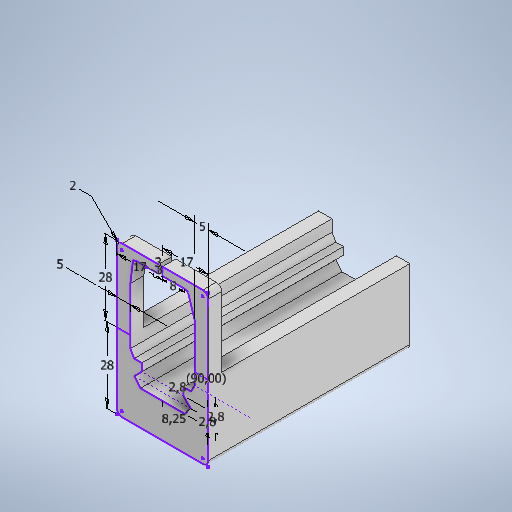
# Autodesk Inventor part: CaseV1
Saved by Autodesk Inventor 2025.2 (Build 292293000, 293)
## iProperties
Created: 2026-03-06
Part Number: CaseV1
Material: Genérico
Document SubType Name: Modeling
Designer: Periscopio
Density: 1 g/cm^3
Appearance: Valor por defecto
Author: Periscopio
Autodesk Inventor part; units mm, degrees
ref_plane "YZ Plane" through (0, 0, 0) normal (1, 0, 0) x (0, 1, 0)
ref_plane "XZ Plane" through (0, 0, 0) normal (0, 1, 0) x (-1, 0, 0)
ref_plane "XY Plane" through (0, 0, 0) normal (0, 0, 1) x (1, 0, 0)
sketch "Boceto1" plane through (0, 0, 0) normal (0, 0, 1) x (1, 0, 0)
  line L0 (0, 0) -> (8.25, 0)
  line L1 (-10.5, 2.8) -> (10.5, 2.8) construction
  line L2 (-7.75, 5.6) -> (7.75, 5.6) construction
  line L3 (10.5, 2.8) -> (8.25, 0)
  line L4 (7.75, 5.6) -> (10.5, 2.8)
  line L5 (7.75, 5.6) -> (7.75, 8.4)
  line L6 (7.75, 8.4) -> (10.55, 8.4)
  line L7 (11.95, 10.9) -> (10.55, 8.4)
  line L8 (11.95, 10.9) -> (11.95, 31.9)
  line L9 (11.95, 10.9) -> (32.95, 10.9) construction
  line L10 (9.4, 39.9) -> (11.95, 31.9)
  line L11 (9.4, 39.9) -> (9.75, 39.9) construction
  line L12 (2.95, 40.25) -> (5.95, 40.25) construction
  line L13 (0, 43.25) -> (-0.05, 43.25)
  line L14 (-3.05, 43.25) -> (-0.05, 43.25) construction
  line L15 (-0.05, 43.25) -> (-0.05, 40.25)
  line L16 (-0.05, 40.25) -> (7.95, 40.25)
  line L17 (7.95, 40.25) -> (9.4, 39.9)
  line L18 (0, 0) -> (-8.25, 0)
  line L19 (-10.5, 2.8) -> (-8.25, 0)
  line L20 (-7.75, 5.6) -> (-10.5, 2.8)
  line L21 (-7.75, 5.6) -> (-7.75, 8.4)
  line L22 (-7.75, 8.4) -> (-10.6, 8.4)
  line L23 (-12, 10.9) -> (-10.6, 8.4)
  line L24 (-12, 10.9) -> (-12, 31.9)
  line L25 (-11, 39.9) -> (-12, 31.9)
  line L26 (-11, 39.9) -> (-11.35, 39.9) construction
  line L27 (0, 43.25) -> (-1.5, 43.25)
  line L28 (-1.55, 43.25) -> (-1.55, 40.25)
  line L29 (-1.55, 40.25) -> (-9.55, 40.25)
  line L30 (-9.55, 40.25) -> (-11, 39.9)
  line L31 (-3.5, 43.25) -> (-1.5, 43.25) construction
  line L32 (0, 43.25) -> (-15, 43.25)
  line L33 (-17, 41.25) -> (-17, 15.25)
  line L34 (-17, 15.25) -> (-12, 15.25)
  line L35 (-17, 15.25) -> (-17, -10.75)
  line L36 (-15, -12.75) -> (0, -12.75)
  line L37 (16.95, 41.25) -> (16.95, 15.25)
  line L38 (16.95, 15.25) -> (11.9, 15.25)
  line L39 (16.95, 15.25) -> (16.95, -10.75)
  line L40 (14.95, -12.75) -> (0, -12.75)
  line L41 (14.95, 43.25) -> (-0.05, 43.25)
  arc A0 (-15, 43.25) -> (-17, 41.25) centre (-15, 41.25) ccw
  arc A1 (16.95, 41.25) -> (14.95, 43.25) centre (14.95, 41.25) ccw
  arc A2 (14.95, -12.75) -> (16.95, -10.75) centre (14.95, -10.75) ccw
  arc A3 (-17, -10.75) -> (-15, -12.75) centre (-15, -10.75) ccw
  point P0 (-5.95, 40.25)
  point P1 (-0.05, 43.25)
  point P2 (-17, 43.25)
  point P3 (16.95, 43.25)
  point P4 (-17, -12.75)
  point P5 (16.95, -12.75)
  point P6 (11.95, 15.25)
  point P7 (-1.55, 43.25)
  dimension "d40" = 2.8
  dimension "d45" = 90
  dimension "d52" = 8.25
  dimension "d53" = 2.8
  dimension "d54" = 2.8
  dimension "d61" = 3
  dimension "d63" = 3
  dimension "d65" = 8
  dimension "d71" = 17
  dimension "d73" = 28
  dimension "d74" = 28
  dimension "d79" = 17
  dimension "d80" = 5
  dimension "d81" = 5
  dimension "d82" = 2
  constraints: 84 end point, 9 point on line, 8 horizontal, 8 perpendicular, 8 point on circle, 8 tangent, 4 centre point, 4 vertical, 3 equal radius
  measures "d40" distance of L2.end L5.end
  measures "d45" angle of L9 L8
  measures "d52" distance of L0.start L0.end
  measures "d53" vertical distance of L1.end L3.end
  measures "d54" vertical distance of L2.end L1.end
  measures "d61" distance of L14.start L13.end
  measures "d63" distance of L14.end L15.end
  measures "d65" distance of L15.end L16.end
  measures "d71" distance of L13.start point (-17, 43.25)
  measures "d73" distance of point (-17, 43.25) L33.end
  measures "d74" distance of L33.end point (-17, -12.75)
  measures "d79" distance of point (16.95, 43.25) L14.end
  measures "d80" distance between parallel lines of L33 L24
  measures "d81" distance between parallel lines of L37 L8
  measures "d82" radius of A0
extrude "Extrusión2" add sketch "Boceto1" against normal blind 5 contours L8 L10 L17 L16 L15 L13 L41 A1 L37 L38 | L34 L33 A0 L32 L28 L29 L30 L25 L24
extrude "Extrusión3" add sketch "Boceto1" against normal blind 75 contours L0 L3 L4 L5 L6 L7 L8 L38 L39 A2 L40 L36 A3 L35 L34 L24 L23 L22 L21 L20 L19 L18
